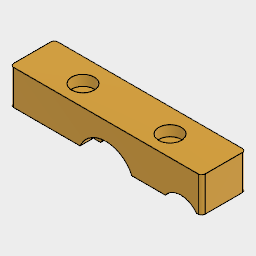
Retainer_F01 (Autodesk Fusion 360 design; units mm, degrees)
Autodesk Fusion 360 part; units mm, degrees
sketch "スケッチ1" plane through (0, 0, 0) normal (0, 0, 1) x (1, 0, 0)
  line L0 (-27.5, 6.35) -> (27.5, 6.35)
  line L1 (27.5, 6.35) -> (27.5, -6.35)
  line L2 (27.5, -6.35) -> (-27.5, -6.35)
  line L3 (-27.5, -6.35) -> (-27.5, 6.35)
  line L4 (-27.5, 6.35) -> (27.5, -6.35) construction
  line L5 (27.5, 6.35) -> (-27.5, -6.35) construction
  circle A0 centre (-12.5, -0.425) radius 1.75
  circle A1 centre (12.5, -0.425) radius 1.75
  dimension "d1" = 55
  dimension "d2" = 12.7
  dimension "d3" = 3.5
  dimension "d4" = 3.5
  dimension "d5" = 15
  dimension "d6" = 15
  dimension "d7" = 5.925
  dimension "d8" = 5.925
  measures "d1" distance of L1.end L2.end
  measures "d2" distance of L0.end L1.end
  measures "d3" diameter of A0
  measures "d4" diameter of A1
  measures "d5" distance of L3 A0.centre
  measures "d6" distance of L1 A1.centre
  measures "d7" distance of L2 A1.centre
  measures "d8" distance of L2 A0.centre
extrude "押し出し1" add sketch "スケッチ1" along normal blind 10 contours L0 L1 L2 L3 | A0 | A1
extrude "押し出し2" cut sketch "スケッチ1" along normal blind 6.6 contours A0 | A1
sketch "スケッチ2" plane through (0, 0, 10) normal (0, 0, 1) x (-1, 0, 0)
  line L0 (27.5, 6.35) -> (-27.5, 6.35)
  line L1 (-27.5, 6.35) -> (-27.5, -6.35)
  line L2 (-27.5, -6.35) -> (27.5, -6.35)
  line L3 (27.5, -6.35) -> (27.5, 6.35)
  circle A0 centre (12.5, 0.425) radius 3.25
  circle A1 centre (-12.5, 0.425) radius 3.25
  point P0 (12.5, 0.425)
  point P1 (-12.5, 0.425)
  dimension "d13" = 6.5
  dimension "d14" = 6.5
  measures "d13" diameter of A0
  measures "d14" diameter of A1
extrude "押し出し3" cut sketch "スケッチ2" against normal blind 3 contours A0 | A1
sketch "スケッチ3" plane through (0, 6.35, 0) normal (0, 1, 0) x (-1, 0, 0)
  line L0 (-27.5, 0) -> (27.5, 0)
  line L1 (27.5, 0) -> (27.5, 10)
  line L2 (27.5, 10) -> (-27.5, 10)
  line L3 (-27.5, 10) -> (-27.5, 0)
  circle A0 centre (0, -3.25) radius 8.1
  circle A1 centre (0, -3.25) radius 6.25
  line L4 (27.5, 0) -> (-27.5, 0)
  circle A2 centre (-21.5, -3.25) radius 5.5
  dimension "d17" = 16.2
  dimension "d18" = 12.5
  dimension "d19" = 3.25
  dimension "d20" = 11
  dimension "d21" = 3.25
  dimension "d22" = 6
  measures "d17" diameter of A0
  measures "d18" diameter of A1
  measures "d19" distance of A0.centre L4
  measures "d20" diameter of A2
  measures "d21" distance of L4 A2.centre
  measures "d22" distance of L3 A2.centre
extrude "押し出し4" cut sketch "スケッチ3" against normal through all contours L0 L4 A2 | L0 A1 L4 picked at (-20.9476, 1.4676) picked at (-0.812, 1.6265)
extrude "押し出し5" cut sketch "スケッチ3" against normal blind 4 contours L0 A0 A1 L4 picked at (-6.5437, 0.3454)
extrude "押し出し6" cut sketch "スケッチ3" against normal up to surface (3.8 mm away) from surface at -8.9 contours L0 A0 A1 L4 picked at (-6.5437, 0.3454)
fillet "フィレット1" radius 1 4 edges at (-27.5, -6.35, 5) (-27.5, 6.35, 5) (27.5, -6.35, 5) (27.5, 6.35, 5)
equation "d8 = d7"
